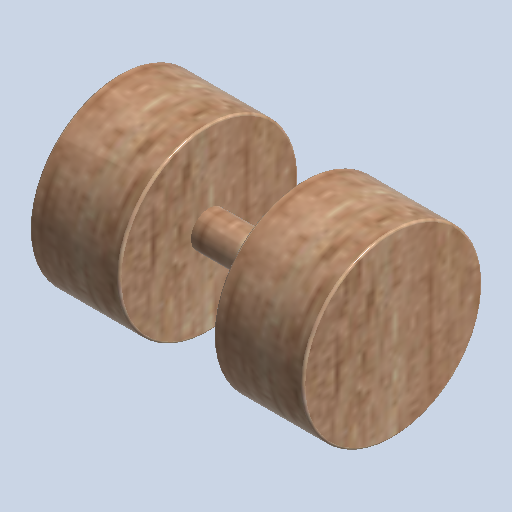
# Autodesk Inventor part: kola
Saved by Autodesk Inventor 2025.2 (Build 292293000, 293)
## iProperties
Part Number: kola
Material: Wood (Birch)
Document SubType Name: Modeling
Designer: fanda
Appearance: Birch - Natural Polished
Density: 0.55 g/cm^3
Author: fanda
Autodesk Inventor part; units mm, degrees
ref_plane "YZ Plane" through (0, 0, 0) normal (1, 0, 0) x (0, 1, 0)
ref_plane "XZ Plane" through (0, 0, 0) normal (0, 1, 0) x (-1, 0, 0)
ref_plane "XY Plane" through (0, 0, 0) normal (0, 0, 1) x (1, 0, 0)
sketch "Sketch1" plane through (0, 0, 0) normal (0, 0, 1) x (1, 0, 0)
  line L0 (-10.1298, 1.8234) -> (50.8702, 1.8234)
  line L1 (-10.1298, 1.8234) -> (-10.1298, 21.3234)
  line L2 (-9.6298, 21.8234) -> (9.3702, 21.8234)
  line L3 (9.8702, 21.3234) -> (9.8702, 1.8234)
  line L4 (9.8702, 1.8234) -> (9.8702, 5.8234)
  line L5 (9.8702, 5.8234) -> (30.8702, 5.8234)
  line L6 (30.8702, 5.8234) -> (30.8702, 1.8234)
  line L7 (30.8702, 1.8234) -> (30.8702, 21.3234)
  line L8 (31.3702, 21.8234) -> (50.3702, 21.8234)
  line L9 (50.8702, 21.3234) -> (50.8702, 1.8234)
  arc A0 (-9.6298, 21.8234) -> (-10.1298, 21.3234) centre (-9.6298, 21.3234) ccw
  arc A1 (9.8702, 21.3234) -> (9.3702, 21.8234) centre (9.3702, 21.3234) ccw
  arc A2 (31.3702, 21.8234) -> (30.8702, 21.3234) centre (31.3702, 21.3234) ccw
  arc A3 (50.8702, 21.3234) -> (50.3702, 21.8234) centre (50.3702, 21.3234) ccw
  point P0 (0, 0)
  point P1 (-10.1298, 21.8234)
  point P2 (9.8702, 21.8234)
  point P3 (30.8702, 21.8234)
  point P4 (50.8702, 21.8234)
  dimension "d0" = 61
  dimension "d1" = 20
  dimension "d2" = 20
  dimension "d3" = 4
  dimension "d4" = 21
  dimension "d5" = 20
  dimension "d7" = 0.5
  dimension "d8" = 0.5
  constraints: 20 end point, 12 point on line, 8 point on circle, 8 tangent, 4 centre point, 3 horizontal, 3 perpendicular, 2 equal radius, 1 vertical
  measures "d0" distance of L0.start L0.end
  measures "d1" distance of L0.start point (-10.13, 21.823)
  measures "d2" distance of point (-10.13, 21.823) point (9.87, 21.823)
  measures "d3" distance of L3.end L4.end
  measures "d4" distance of L4.end L5.end
  measures "d5" distance of point (30.87, 21.823) point (50.87, 21.823)
  measures "d7" radius of A0
  measures "d8" radius of A1
revolve "Revolution1" add sketch "Sketch1" angle 360 about axis through (-10.1298, 1.8234, 0) along (1, 0, 0)
